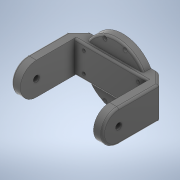
# Autodesk Inventor part: servo_arm
Saved by Autodesk Inventor 2020 (Build 240168000, 168)
## iProperties
Created: 2020-06-27
Part Number: servo_arm
Material: アセタール樹脂、黒
Document SubType Name: Modeling
Designer: haya
Density: 1.425 g/cm^3
Appearance: 滑らか - 黒
Author: haya
Autodesk Inventor part; units mm, degrees
ref_plane "YZ Plane" through (0, 0, 0) normal (1, 0, 0) x (0, 1, 0)
ref_plane "XZ Plane" through (0, 0, 0) normal (0, 1, 0) x (-1, 0, 0)
ref_plane "XY Plane" through (0, 0, 0) normal (0, 0, 1) x (1, 0, 0)
sketch "スケッチ1" plane through (0, 0, 0) normal (0, 0, 1) x (1, 0, 0)
  circle A0 centre (0, 0) radius 16
  dimension "d0" = 32
  constraints: 1 centre point, 1 coincident
  measures "d0" diameter of A0
extrude "押し出し1" add sketch "スケッチ1" along normal blind 4
sketch "スケッチ2" plane through (0, 0, 0) normal (0, 0, -1) x (-1, 0, 0)
  line L0 (-22.75, 8) -> (22.75, 8)
  line L1 (22.75, 8) -> (22.75, -8)
  line L2 (22.75, -8) -> (-22.75, -8)
  line L3 (-22.75, -8) -> (-22.75, 8)
  line L4 (0, 0) -> (0, 8)
  line L5 (0, 0) -> (22.75, 0)
  dimension "d3" = 45.5
  dimension "d4" = 16
  constraints: 12 end point, 3 perpendicular, 2 midpoint, 2 parallel, 1 horizontal, 2 other
  measures "d3" distance of L0.start L0.end
  measures "d4" distance of L0.end L1.end
extrude "押し出し2" add sketch "スケッチ2" against normal blind 6
sketch "スケッチ3" plane through (0, 0, 0) normal (0, 0, -1) x (-1, 0, 0)
  line L0 (22.75, -8) -> (-22.75, -8) projected
  line L1 (-22.75, 8) -> (22.75, 8) projected
  line L2 (-22.75, -8) -> (-18.25, -8)
  line L3 (-18.25, -8) -> (-18.25, 8)
  line L4 (-18.25, 8) -> (-22.75, 8)
  line L5 (-22.75, 8) -> (-22.75, -8)
  line L6 (22.75, 8) -> (13.8564, 8) projected
  line L7 (22.75, -8) -> (18.25, -8)
  line L8 (18.25, -8) -> (18.25, 8)
  line L9 (18.25, 8) -> (22.75, 8)
  line L10 (22.75, 8) -> (22.75, -8)
  point P0 (0, 0)
  point P1 (22.75, 8)
  dimension "d7" = 4.5
  dimension "d8" = 4.5
  constraints: 16 end point, 4 parallel, 2 horizontal, 2 perpendicular, 2 point on line
  measures "d7" distance between parallel lines of L3 L5
  measures "d8" distance between parallel lines of L8 L10
extrude "押し出し3" add sketch "スケッチ3" against normal blind 25 contours L0 L8 L1 L10 | L0 L5 L1 L3
sketch "スケッチ4" plane through (22.75, -8, 0) normal (1, 0, 0) x (0, 0, -1)
  line L0 (-25, 16) -> (-25, 0) projected
  circle A0 centre (-25, 8) radius 8
  point P0 (0, 8)
  point P1 (-25, 0)
  constraints: 1 midpoint, 3 other
extrude "押し出し4" add sketch "スケッチ4" against normal up to surface (4.5 mm away) contours L0 A0 picked at (-27.6472, 7.6786)
sketch "スケッチ5" plane through (-22.75, -8, 0) normal (-1, 0, 0) x (0, 0, 1)
  line L0 (25, 16) -> (25, 0) projected
  line L1 (6, 0) -> (25, 0) projected
  circle A0 centre (25, 8) radius 8
  point P0 (0, 8)
  constraints: 1 midpoint, 3 other
extrude "押し出し5" add sketch "スケッチ5" against normal up to surface (4.5 mm away) contours A0 L0 picked at (27.5998, 8.5934)
sketch "スケッチ6" plane through (0, 0, 0) normal (0, 0, -1) x (-1, 0, 0)
  line L0 (0, 0) -> (0, 16)
  arc A0 (13.8564, 8) -> (-13.8564, 8) centre (0, 0) ccw projected
  line L1 (0, 0) -> (25.566, 0)
  point P0 (5, 13.5)
  point P1 (-5, 13.5)
  point P2 (5, -13.5)
  point P3 (-5, -13.5)
  dimension "d15" = 10
  dimension "d16" = 27
  constraints: 4 end point, 3 symmetric about line, 1 horizontal, 1 point on circle, 1 vertical
  measures "d15" distance of point (5, 13.5) point (-5, 13.5)
  measures "d16" distance of point (-5, -13.5) point (-5, 13.5)
hole "穴1" at (-5, -13.5, 0) at (5, -13.5, 0) at (5, 13.5, 0) at (-5, 13.5, 0) direction (0, 0, 1) diameter 2.1 depth 8 tip angle 118
sketch "スケッチ8" plane through (22.75, -8, 0) normal (1, 0, 0) x (0, 0, -1)
  line L0 (0, 16) -> (0, 0) projected
  line L1 (0, 16) -> (-25, 16) projected
  point P0 (0, 8)
  point P1 (-25, 8)
  dimension "d24" = 25
  dimension "d25" = 8
  measures "d24" distance from line of point (-25, 8) L0
  measures "d25" distance from line of L1 point (-25, 8)
hole "穴2" at (22.75, 0, 25) direction (-1, 0, 0) diameter 3 end through all
sketch "スケッチ9" plane through (0, 0, 0) normal (0, 0, -1) x (-1, 0, 0)
  line L0 (0, 0) -> (0, 16)
  arc A0 (13.8564, 8) -> (-13.8564, 8) centre (0, 0) ccw projected
  line L1 (0, 0) -> (22.75, 0)
  line L2 (22.75, -8) -> (22.75, 8) projected
  point P0 (13.5, 5)
  point P1 (13.5, -5)
  point P2 (-13.5, 5)
  point P3 (-13.5, -5)
  dimension "d33" = 10
  dimension "d34" = 27
  constraints: 4 end point, 3 symmetric about line, 1 coincident, 1 horizontal, 1 midpoint, 1 point on circle, 1 vertical
  measures "d33" distance of point (-13.5, -5) point (-13.5, 5)
  measures "d34" distance of point (13.5, 5) point (-13.5, 5)
hole "穴3" at (-13.5, 5, 0) at (-13.5, -5, 0) at (13.5, 5, 0) at (13.5, -5, 0) direction (0, 0, 1) diameter 1.567 end through all thread size "M2x0.4" class "6H" standard "ISO Metric profile"
chamfer "面取り1" distance 5 angle 45 2 edges at (22.75, 0, 0) (-22.75, 0, 0)
fillet "フィレット1" radius 1 14 edges at (22.75, 0, 33) (22.75, -8, 15) (22.75, 8, 15) (-22.75, 0, 33) (-22.75, -8, 15) (-22.75, 8, 15) (0, 8, 6) (0, -8, 6) (0, -16, 4) (0, 16, 4) (20.25, 8, 2.5) (20.25, -8, 2.5) (-20.25, 8, 2.5) (-20.25, -8, 2.5)
